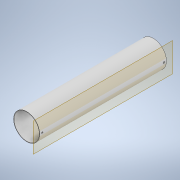
# Autodesk Inventor part: Segment_elektro
Saved by Autodesk Inventor 2020 (Build 240168000, 168)
## iProperties
Created: 2022-01-25
Part Number: Segment_elektro
Material: Generisch
Document SubType Name: Modeling
Designer: sp
Density: 1 g/cm^3
Appearance: Vorgabe
Author: sp
Autodesk Inventor part; units mm, degrees
ref_plane "XZ Plane" through (0, 0, 0) normal (0, 1, 0) x (-1, 0, 0)
ref_plane "XY Plane" through (0, 0, 0) normal (0, 0, 1) x (1, 0, 0)
sketch "Skizze1" plane through (0, 0, 0) normal (0, 0, 1) x (1, 0, 0)
  circle A0 centre (0, 0) radius 31
  circle A1 centre (0, 0) radius 30
  dimension "d0" = 62
  dimension "d1" = 60
  constraints: 2 centre point, 2 coincident
  measures "d0" diameter of A0
  measures "d1" diameter of A1
extrude "Extrusion1" add sketch "Skizze1" along normal mid plane 300
ref_plane "Arbeitsebene1" through (30.5, 0, 0) normal (1, 0, 0) x (0, 1, 0)
sketch "Skizze2" plane through (30.5, 0, 0) normal (1, 0, 0) x (0, 1, 0)
  circle A0 centre (0, 144) radius 1.75
  line L0 (31, 150) -> (-31, 150) projected
  point P0 (0, 0)
  dimension "d5" = 3.5
  dimension "d6" = 6
  constraints: 1 centre point
  measures "d5" diameter of A0
  measures "d6" distance from line of L0 A0.centre
extrude "Extrusion2" cut sketch "Skizze2" against normal mid plane 10
mirror "Spiegeln1" about plane through (0, 0, 0) normal (0, 0, 1) of "Extrusion2"
